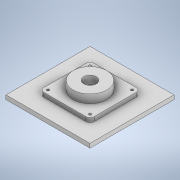
# Autodesk Inventor part: Base Plate 2
Saved by Autodesk Inventor 2020 (Build 240168000, 168)
## iProperties
Created: 2022-02-16
Part Number: Base Plate 2
Material: Generic
Document SubType Name: Modeling
Designer: New-Computer
Density: 1 g/cm^3
Appearance: Default
Author: New-Computer
Autodesk Inventor part; units mm, degrees
ref_plane "YZ Plane" through (0, 0, 0) normal (1, 0, 0) x (0, 1, 0)
ref_plane "XZ Plane" through (0, 0, 0) normal (0, 1, 0) x (-1, 0, 0)
ref_plane "XY Plane" through (0, 0, 0) normal (0, 0, 1) x (1, 0, 0)
sketch "Sketch1" plane through (0, 0, 0) normal (0, 1, 0) x (-1, 0, 0)
  line L0 (-100, 100) -> (100, 100)
  line L1 (100, 100) -> (100, -100)
  line L2 (100, -100) -> (-100, -100)
  line L3 (-100, -100) -> (-100, 100)
  line L4 (-100, 100) -> (100, -100) construction
  line L5 (100, 100) -> (-100, -100) construction
  point P0 (0, 0)
  dimension "d0" = 200
  dimension "d1" = 200
  constraints: 12 end point, 2 midpoint, 2 parallel, 1 horizontal, 1 perpendicular
  measures "d0" distance between parallel lines of L2 L0
  measures "d1" distance between parallel lines of L3 L1
extrude "Extrusion1" add sketch "Sketch1" along normal blind 10
sketch "Sketch2" plane through (0, 10, 0) normal (0, 1, 0) x (1, 0, 0)
  line L0 (60, -60) -> (-60, -60)
  line L1 (-60, -60) -> (-60, 60)
  line L2 (-60, 60) -> (60, 60)
  line L3 (60, 60) -> (60, -60)
  line L4 (60, -60) -> (-60, 60) construction
  line L5 (-60, -60) -> (60, 60) construction
  point P0 (0, 0)
  dimension "d4" = 120
  dimension "d5" = 120
  constraints: 12 end point, 2 midpoint, 2 parallel, 1 horizontal, 1 perpendicular
  measures "d4" distance between parallel lines of L3 L1
  measures "d5" distance between parallel lines of L2 L0
extrude "Extrusion2" add sketch "Sketch2" along normal blind 10
fillet "Fillet1" radius 10 4 edges at (60, 15, 60) (60, 15, -60) (-60, 15, 60) (-60, 15, -60)
sketch "Sketch3" plane through (0, 20, 0) normal (0, 1, 0) x (1, 0, 0)
  circle A0 centre (0, 0) radius 15
  circle A1 centre (0, 0) radius 40
  dimension "d9" = 30
  dimension "d19" = 80
  constraints: 2 centre point, 2 coincident
  measures "d9" diameter of A0
  measures "d19" diameter of A1
extrude "Extrusion3" add sketch "Sketch3" along normal blind 20
sketch "Sketch4" plane through (0, 20, 0) normal (0, 1, 0) x (1, 0, 0)
  arc A0 (60, 50) -> (50, 60) centre (50, 50) ccw projected
  arc A1 (50, -60) -> (60, -50) centre (50, -50) ccw projected
  arc A2 (-60, -50) -> (-50, -60) centre (-50, -50) ccw projected
  arc A3 (-50, 60) -> (-60, 50) centre (-50, 50) ccw projected
  point P0 (0, 0)
  constraints: 4 coincident
hole "Hole1" at (50, 20, 50) at (-50, 20, 50) at (50, 20, -50) at (-50, 20, -50) direction (0, -1, 0) diameter 6 end through all
body "Solid1"
